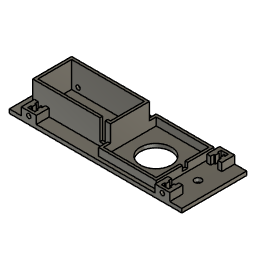
Cont Mtr Lower Case v1 (Autodesk Fusion 360 design; units mm, degrees)
Autodesk Fusion 360 part; units mm, degrees
sketch "Sketch1" plane through (0, 0, 0) normal (0, 0, 1) x (1, 0, 0)
  line L0 (0, 0) -> (60, 0)
  line L1 (60, 0) -> (60, 30)
  line L2 (60, 30) -> (0, 30)
  line L3 (0, 30) -> (0, 0)
  dimension "d1" = 60
  dimension "d2" = 30
  constraint horizontal L0
  constraint vertical L1
  constraint horizontal L2
  constraint vertical L3
  constraint coincident L0.start L3.end
  measures "d1" distance of L0.start L0.end
  measures "d2" distance of L0.start L2.end
extrude "Extrude1" add sketch "Sketch1" along normal blind 22
sketch "Sketch2" plane through (0, 0, 22) normal (0, 0, 1) x (-1, 0, 0)
  line L0 (0, -30) -> (0, 0)
  line L1 (0, 0) -> (-60, 0)
  line L2 (-60, 0) -> (-60, -30)
  line L3 (-60, -30) -> (0, -30)
  line L4 (-2, -28) -> (-58, -28)
  line L5 (-58, -28) -> (-58, -2)
  line L6 (-58, -2) -> (-2, -2)
  line L7 (-2, -2) -> (-2, -28)
  dimension "d5" = 56
  dimension "d6" = 26
  dimension "d7" = 2
  dimension "d8" = 2
  constraint horizontal L4
  constraint vertical L5
  constraint horizontal L6
  constraint vertical L7
  measures "d5" distance of L4.start L4.end
  measures "d6" distance of L4.start L6.end
  measures "d7" distance of L3 L4
  measures "d8" distance of L0 L7
extrude "Extrude2" cut sketch "Sketch2" against normal blind 20 contours L4 L5 L6 L7
sketch "Sketch3" plane through (0, 0, 0) normal (0, -1, 0) x (1, 0, 0)
  line L0 (0, 0) -> (60, 0)
  line L1 (60, 0) -> (60, 22)
  line L2 (60, 22) -> (0, 22)
  line L3 (0, 22) -> (0, 0)
  line L4 (0, 0) -> (60, 0)
  line L5 (60, 0) -> (60, 3)
  line L6 (60, 3) -> (0, 3)
  line L7 (0, 3) -> (0, 0)
  dimension "d11" = 60
  dimension "d12" = 3
  constraint horizontal L4
  constraint vertical L5
  constraint horizontal L6
  constraint vertical L7
  constraint coincident L0.start L3.end
  measures "d11" distance of L0.start L0.end
  measures "d12" distance of L0.start L6.end
extrude "Extrude3" add sketch "Sketch3" along normal blind 8 contours L0 L1 L3 L4 L5 L6 L7
sketch "Sketch4" plane through (0, 30, 0) normal (0, 1, 0) x (-1, 0, 0)
  line L0 (-60, 0) -> (0, 0)
  line L1 (0, 0) -> (0, 22)
  line L2 (0, 22) -> (-60, 22)
  line L3 (-60, 22) -> (-60, 0)
  line L4 (-60, 0) -> (0, 0)
  line L5 (0, 0) -> (0, 3)
  line L6 (0, 3) -> (-60, 3)
  line L7 (-60, 3) -> (-60, 0)
  dimension "d15" = 3
  constraint horizontal L4
  constraint vertical L5
  constraint horizontal L6
  constraint vertical L7
  constraint coincident L0.start L3.end
  measures "d15" distance of L0.start L6.end
extrude "Extrude4" add sketch "Sketch4" along normal blind 8 contours L0 L1 L3 L4 L5 L6 L7
sketch "Sketch5" plane through (60, 0, 0) normal (1, 0, 0) x (0, 1, 0)
  line L0 (-8, 0) -> (38, 0)
  line L1 (38, 0) -> (38, 3)
  line L2 (38, 3) -> (30, 3)
  line L3 (30, 3) -> (30, 22)
  line L4 (30, 22) -> (0, 22)
  line L5 (0, 22) -> (0, 3)
  line L6 (0, 3) -> (-8, 3)
  line L7 (-8, 3) -> (-8, 0)
  line L8 (-8, 3) -> (38, 3)
  line L9 (38, 3) -> (38, 0)
  line L10 (38, 0) -> (-8, 0)
  line L11 (-8, 0) -> (-8, 3)
  constraint horizontal L8
  constraint vertical L9
  constraint horizontal L10
  constraint vertical L11
  constraint coincident L0.end L1.start
  constraint coincident L6.end L7.start
extrude "Extrude5" add sketch "Sketch5" along normal blind 50 contours L0 L1 L2 L6 L7 L8 L9 L10 L11
sketch "Sketch6" plane through (0, 0, 0) normal (-1, 0, 0) x (0, -1, 0)
  line L0 (-38, 0) -> (8, 0)
  line L1 (8, 0) -> (8, 3)
  line L2 (8, 3) -> (0, 3)
  line L3 (0, 3) -> (0, 22)
  line L4 (0, 22) -> (-30, 22)
  line L5 (-30, 22) -> (-30, 3)
  line L6 (-30, 3) -> (-38, 3)
  line L7 (-38, 3) -> (-38, 0)
  line L8 (-38, 3) -> (8, 3)
  line L9 (8, 3) -> (8, 0)
  line L10 (8, 0) -> (-38, 0)
  line L11 (-38, 0) -> (-38, 3)
  constraint horizontal L8
  constraint vertical L9
  constraint horizontal L10
  constraint vertical L11
  constraint coincident L0.end L1.start
  constraint coincident L6.end L7.start
extrude "Extrude6" add sketch "Sketch6" along normal blind 8 contours L0 L1 L2 L6 L7 L8 L9 L10 L11
sketch "Sketch7" plane through (0, 0, 3) normal (0, 0, 1) x (-1, 0, 0)
  line L0 (8, 8) -> (-110, 8)
  line L1 (-110, 8) -> (-110, -38)
  line L2 (-110, -38) -> (8, -38)
  line L3 (8, -38) -> (8, 8)
  line L4 (0, 0) -> (0, -30)
  line L5 (0, -30) -> (-60, -30)
  line L6 (-60, -30) -> (-60, 0)
  line L7 (-60, 0) -> (0, 0)
  line L8 (-60.1, -35.15) -> (-100.4, -35.15) construction
  line L9 (-100.4, -35.15) -> (-100.4, 5.15) construction
  line L10 (-100.4, 5.15) -> (-60.1, 5.15) construction
  line L11 (-60.1, 5.15) -> (-60.1, -35.15) construction
  line L12 (-60, -15) -> (-127.1, -15) construction
  line L13 (-100.5, -35.25) -> (-60, -35.25)
  line L14 (-60, -35.25) -> (-60, 5.25)
  line L15 (-60, 5.25) -> (-100.5, 5.25)
  line L16 (-100.5, 5.25) -> (-100.5, -35.25)
  line L17 (-58, -37.25) -> (-58, 7.25)
  line L18 (-58, 7.25) -> (-102.5, 7.25)
  line L19 (-102.5, 7.25) -> (-102.5, -37.25)
  line L20 (-102.5, -37.25) -> (-58, -37.25)
  dimension "d22" = 40.3
  dimension "d23" = 40.3
  dimension "d24" = 20.15
  dimension "d25" = 0.1
  dimension "d31" = 40.5
  dimension "d32" = 40.5
  dimension "d33" = 68
  dimension "d34" = 20.25
  dimension "d35" = 2
  constraint horizontal L8
  constraint vertical L9
  constraint horizontal L10
  constraint vertical L11
  constraint midpoint L6 L12.start
  constraint perpendicular L1 L12
  constraint horizontal L13
  constraint vertical L14
  constraint horizontal L15
  constraint vertical L16
  measures "d22" distance of L8.start L8.end
  measures "d23" distance of L8.start L10.end
  measures "d24" distance of L8 L12
  measures "d25" distance of L6 L11
  measures "d31" distance of L13.start L13.end
  measures "d32" distance of L13.start L15.end
  measures "d33" distance of L3 L14
  measures "d34" distance of L12 L13
move_face "OffsetFaces1" offset 2 1 faces at (70.6667, 38, 2)
extrude "Extrude7" add 1 faces at (31.3333, -8, 2) along direction (0, -1, 0) blind 2
extrude "Extrude8" add 1 faces at (110, 23.3333, 1) along direction (1, 0, 0) blind 15
extrude "Extrude9" add sketch "Sketch7" along normal blind 6 contours L5 L7 L13 L14 L15 L16 L17 L18 L19 L20
sketch "Sketch9" plane through (0, 0, 3) normal (0, 0, 1) x (-1, 0, 0)
  line L0 (-60, -35.25) -> (-60, 5.25)
  line L1 (-60, 5.25) -> (-100.5, 5.25)
  line L2 (-100.5, 5.25) -> (-100.5, -35.25)
  line L3 (-100.5, -35.25) -> (-60, -35.25)
  circle A0 centre (-80, -15) radius 12
  dimension "d38" = 24
  measures "d38" diameter of A0
extrude "Extrude10" cut sketch "Sketch9" against normal blind 12 contours A0
sketch "Sketch10" plane through (0, 0, 9) normal (0, 0, 1) x (-1, 0, 0)
  line L0 (-60, 0) -> (-58, 0)
  line L1 (-58, 0) -> (-58, 7.25)
  line L2 (-58, 7.25) -> (-102.5, 7.25)
  line L3 (-102.5, 7.25) -> (-102.5, -37.25)
  line L4 (-102.5, -37.25) -> (-58, -37.25)
  line L5 (-58, -37.25) -> (-58, -30)
  line L6 (-58, -30) -> (-60, -30)
  line L7 (-60, -30) -> (-60, -35.25)
  line L8 (-60, -35.25) -> (-100.5, -35.25)
  line L9 (-100.5, -35.25) -> (-100.5, 5.25)
  line L10 (-100.5, 5.25) -> (-60, 5.25)
  line L11 (-60, 5.25) -> (-60, 0)
  line L12 (-100.5, -16.9697) -> (-102.5, -16.9697)
  line L13 (-102.5, -16.9697) -> (-102.5, -12.9697)
  line L14 (-102.5, -12.9697) -> (-100.5, -12.9697)
  line L15 (-100.5, -12.9697) -> (-100.5, -16.9697)
  line L16 (-110, -14.9697) -> (-85, -14.9697) construction
  dimension "d41" = 2
  dimension "d42" = 4
  dimension "d43" = 2
  constraint horizontal L12
  constraint vertical L13
  constraint horizontal L14
  constraint vertical L15
  constraint coincident L9 L12.start
  constraint perpendicular L9 L16
  measures "d41" distance of L12.start L12.end
  measures "d42" distance of L12.start L14.end
  measures "d43" distance of L12 L16
extrude "Extrude11" cut sketch "Sketch10" against normal blind 4 contours L3 L9 L12 L13 L14 L15
sketch "Sketch11" plane through (0, 0, 22) normal (0, 0, 1) x (-1, 0, 0)
  line L0 (-58, -28) -> (-58, -2)
  line L1 (-58, -2) -> (-2, -2)
  line L2 (-2, -2) -> (-2, -28)
  line L3 (-2, -28) -> (-58, -28)
  line L4 (0, -30) -> (0, 0)
  line L5 (0, 0) -> (-60, 0)
  line L6 (-60, 0) -> (-60, -30)
  line L7 (-60, -30) -> (0, -30)
  line L8 (-55.8802, -2) -> (-51.8802, -2)
  line L9 (-51.8802, -2) -> (-51.8802, 0)
  line L10 (-51.8802, 0) -> (-55.8802, 0)
  line L11 (-55.8802, 0) -> (-55.8802, -2)
  dimension "d46" = 4
  constraint horizontal L8
  constraint vertical L9
  constraint horizontal L10
  constraint vertical L11
  constraint coincident L1 L8.start
  measures "d46" distance of L8.start L8.end
extrude "Extrude12" cut sketch "Sketch11" against normal blind 16 contours L1 L5 L8 L9 L10 L11
sketch "Sketch12" plane through (0, 0, 3) normal (0, 0, 1) x (-1, 0, 0)
  line L0 (-58, -30) -> (-58, -37.25)
  line L1 (-58, -37.25) -> (-102.5, -37.25)
  line L2 (-102.5, -37.25) -> (-102.5, 7.25)
  line L3 (-102.5, 7.25) -> (-58, 7.25)
  line L4 (-58, 7.25) -> (-58, 0)
  line L5 (-58, 0) -> (0, 0)
  line L6 (0, 0) -> (0, -30)
  line L7 (0, -30) -> (-58, -30)
  line L8 (-125, -40) -> (8, -40)
  line L9 (8, -40) -> (8, 10)
  line L10 (8, 10) -> (-125, 10)
  line L11 (-125, 10) -> (-125, -40)
  line L12 (-7, -44) -> (-7, 24) construction
  line L13 (-110, -45) -> (-110, 22) construction
  line L14 (-1.25, -30) -> (-1.25, -40)
  line L15 (-1.25, -40) -> (-12.75, -40)
  line L16 (-12.75, -40) -> (-12.75, -30)
  line L17 (-12.75, -30) -> (-9.75, -30)
  line L18 (-9.75, -38) -> (-4.25, -38)
  line L19 (-4.25, -38) -> (-4.25, -30)
  line L20 (-1.25, -30) -> (-4.25, -30)
  line L21 (-9.75, -38) -> (-9.75, -30)
  line L22 (-28.0187, -15) -> (31, -15) construction
  line L23 (-12.75, 0) -> (-9.75, 0)
  line L24 (-12.75, 10) -> (-12.75, 0)
  line L25 (-9.75, 8) -> (-9.75, 0)
  line L26 (-9.75, 8) -> (-4.25, 8)
  line L27 (-4.25, 8) -> (-4.25, 0)
  line L28 (-1.25, 0) -> (-4.25, 0)
  line L29 (-1.25, 0) -> (-1.25, 10)
  line L30 (-1.25, 10) -> (-12.75, 10)
  line L31 (-58.5, 15) -> (-58.5, -52) construction
  line L32 (-104.25, 10) -> (-104.25, 0)
  line L33 (-115.75, 10) -> (-104.25, 10)
  line L34 (-107.25, 8) -> (-112.75, 8)
  line L35 (-107.25, 8) -> (-107.25, 0)
  line L36 (-112.75, 8) -> (-112.75, 0)
  line L37 (-115.75, 0) -> (-115.75, 10)
  line L38 (-115.75, 0) -> (-112.75, 0)
  line L39 (-104.25, 0) -> (-107.25, 0)
  line L40 (-104.25, -30) -> (-107.25, -30)
  line L41 (-107.25, -38) -> (-107.25, -30)
  line L42 (-112.75, -38) -> (-112.75, -30)
  line L43 (-115.75, -30) -> (-112.75, -30)
  line L44 (-115.75, -30) -> (-115.75, -40)
  line L45 (-107.25, -38) -> (-112.75, -38)
  line L46 (-115.75, -40) -> (-104.25, -40)
  line L47 (-104.25, -40) -> (-104.25, -30)
  dimension "d49" = 15
  dimension "d50" = 15
  dimension "d51" = 2.75
  dimension "d52" = 2.75
  dimension "d53" = 3
  dimension "d54" = 3
  dimension "d55" = 2
  dimension "d56" = 66.5
  constraint perpendicular L10 L12
  constraint perpendicular L10 L13
  constraint coincident L7 L14.start
  constraint coincident L8 L14.end
  constraint perpendicular L8 L14
  constraint coincident L8 L15.end
  constraint perpendicular L12 L15
  constraint coincident L7 L16.end
  constraint perpendicular L7 L16
  constraint coincident L7 L17.end
  constraint perpendicular L12 L18
  constraint coincident L7 L19.end
  constraint perpendicular L7 L19
  constraint perpendicular L7 L21
  constraint perpendicular L9 L22
  constraint symmetric L14.start L22 L28.start
  constraint symmetric L14.end L22 L29.end
  constraint symmetric L15.end L22 L24.start
  constraint symmetric L16.end L22 L23.start
  constraint symmetric L17.end L22 L23.end
  constraint symmetric L18.start L22 L25.start
  constraint symmetric L18.end L22 L26.end
  constraint symmetric L19.end L22 L27.end
  constraint vertical L31
  constraint symmetric L14.start L31 L43.start
  constraint symmetric L14.end L31 L44.end
  constraint symmetric L15.end L31 L46.end
  constraint symmetric L16.end L31 L40.start
  constraint symmetric L17.end L31 L40.end
  constraint symmetric L18.start L31 L41.start
  constraint symmetric L18.end L31 L42.start
  constraint symmetric L19.end L31 L42.end
  constraint symmetric L23.start L31 L32.end
  constraint symmetric L23.end L31 L35.end
  constraint symmetric L24.start L31 L32.start
  constraint symmetric L25.start L31 L34.start
  constraint symmetric L26.end L31 L34.end
  constraint symmetric L27.end L31 L36.end
  constraint symmetric L28.start L31 L37.start
  constraint symmetric L29.end L31 L33.start
  measures "d49" distance of L9 L12
  measures "d50" distance of L11 L13
  measures "d51" distance of L12 L19
  measures "d52" distance of L12 L21
  measures "d53" distance of L16 L21
  measures "d54" distance of L14 L19
  measures "d55" distance of L15 L18
  measures "d56" distance of L11 L31
extrude "Extrude13" add sketch "Sketch12" along normal blind 6 contours L7 L8 L14 L15 L16 L17 L18 L19 L20 L21 | L8 L40 L41 L42 L43 L44 L45 L46 L47 | L5 L10 L23 L24 L25 L26 L27 L28 L29 L30 | L10 L32 L33 L34 L35 L36 L37 L38 L39
sketch "Sketch13" plane through (0, -10, 0) normal (0, -1, 0) x (1, 0, 0)
  line L0 (-8, 0) -> (125, 0)
  line L1 (125, 0) -> (125, 3)
  line L2 (125, 3) -> (115.75, 3)
  line L3 (115.75, 3) -> (115.75, 9)
  line L4 (115.75, 9) -> (104.25, 9)
  line L5 (104.25, 9) -> (104.25, 3)
  line L6 (104.25, 3) -> (12.75, 3)
  line L7 (12.75, 3) -> (12.75, 9)
  line L8 (12.75, 9) -> (1.25, 9)
  line L9 (1.25, 9) -> (1.25, 3)
  line L10 (1.25, 3) -> (-8, 3)
  line L11 (-8, 3) -> (-8, 0)
  line L12 (104.25, 3) -> (115.75, 3) construction
  line L13 (103, 8.5) -> (117.6026, 8.5) construction
  line L14 (104.25, 8.5) -> (115.75, 3) construction
  line L15 (115.75, 8.5) -> (104.25, 3) construction
  line L16 (1.25, 3) -> (12.75, 3) construction
  line L17 (-3, 8.5) -> (20, 8.5) construction
  line L18 (1.25, 8.5) -> (12.75, 3) construction
  line L19 (12.75, 8.5) -> (1.25, 3) construction
  point P0 (110, 5.75)
  point P1 (7, 5.75)
  dimension "d59" = 5.5
  dimension "d60" = 5.5
  constraint coincident L5.end L6.start
  constraint coincident L2.end L3.start
  constraint perpendicular L3 L13
  constraint coincident L5 L14.start
  constraint coincident L13 L14.start
  constraint coincident L3 L15.start
  constraint coincident L13 L15.start
  constraint midpoint L15 P0
  constraint coincident L9.end L10.start
  constraint coincident L6.end L7.start
  constraint perpendicular L7 L17
  constraint coincident L9 L18.start
  constraint coincident L17 L18.start
  constraint coincident L7 L19.start
  constraint coincident L17 L19.start
  constraint midpoint L19 P1
  measures "d59" distance of L12 L13
  measures "d60" distance of L16 L17
hole "Hole1" at (7, -10, 5.75) at (110, -10, 5.75) direction (0, 1, 0) diameter 3.3 depth 100 tip angle 118
sketch "Sketch14" plane through (0, 0, 3) normal (0, 0, 1) x (-1, 0, 0)
  line L0 (-9.75, -30) -> (-9.75, -38)
  line L1 (-9.75, -38) -> (-4.25, -38)
  line L2 (-4.25, -38) -> (-4.25, -30)
  line L3 (-4.25, -30) -> (-9.75, -30)
  line L4 (-4.25, -35.5) -> (-9.75, -35.5)
  line L5 (-9.75, -35.5) -> (-9.75, -32.5)
  line L6 (-9.75, -32.5) -> (-4.25, -32.5)
  line L7 (-4.25, -32.5) -> (-4.25, -35.5)
  dimension "d64" = 3
  dimension "d65" = 2.5
  constraint horizontal L4
  constraint vertical L5
  constraint horizontal L6
  constraint vertical L7
  constraint coincident L2 L4.start
  measures "d64" distance of L4.start L6.end
  measures "d65" distance of L1 L4
extrude "Extrude14" add sketch "Sketch14" along normal blind 6 contours L0 L2 L4 L5 L6 L7
sketch "Sketch15" plane through (0, 0, 9) normal (0, 0, 1) x (-1, 0, 0)
  line L0 (-4.25, -35.5) -> (-4.25, -38)
  line L1 (-4.25, -38) -> (-9.75, -38)
  line L2 (-9.75, -38) -> (-9.75, -35.5)
  line L3 (-9.75, -35.5) -> (-4.25, -35.5)
  line L4 (-4.25, -32.5) -> (-9.75, -32.5)
  line L5 (-9.75, -32.5) -> (-9.75, -30)
  line L6 (-9.75, -30) -> (-12.75, -30)
  line L7 (-12.75, -30) -> (-12.75, -40)
  line L8 (-12.75, -40) -> (-1.25, -40)
  line L9 (-1.25, -40) -> (-1.25, -30)
  line L10 (-1.25, -30) -> (-4.25, -30)
  line L11 (-4.25, -30) -> (-4.25, -32.5)
  line L12 (-7, -25.2955) -> (-7, -46) construction
  line L13 (-5.3, -35.5) -> (-8.7, -35.5)
  line L14 (-8.7, -35.5) -> (-8.7, -32.5)
  line L15 (-8.7, -32.5) -> (-5.3, -32.5)
  line L16 (-5.3, -32.5) -> (-5.3, -35.5)
  dimension "d68" = 3.4
  dimension "d69" = 1.7
  dimension "d70" = 5.75
  constraint perpendicular L8 L12
  constraint horizontal L13
  constraint vertical L14
  constraint horizontal L15
  constraint vertical L16
  constraint coincident L3 L13.start
  measures "d68" distance of L13.start L13.end
  measures "d69" distance of L12 L14
  measures "d70" distance of L9 L12
extrude "Extrude15" cut sketch "Sketch15" against normal blind 6 contours L3 L4 L13 L14 L15 L16
sketch "Sketch16" plane through (0, 0, 3) normal (0, 0, 1) x (-1, 0, 0)
  line L0 (-9.75, 8) -> (-9.75, 0)
  line L1 (-9.75, 0) -> (-4.25, 0)
  line L2 (-4.25, 0) -> (-4.25, 8)
  line L3 (-4.25, 8) -> (-9.75, 8)
  line L4 (-7, 2) -> (-7, 16) construction
  line L5 (-1.25, 0) -> (-1.25, 10) construction
  line L6 (-4.25, 2.5) -> (-9.75, 2.5)
  line L7 (-9.75, 2.5) -> (-9.75, 5.5)
  line L8 (-9.75, 5.5) -> (-4.25, 5.5)
  line L9 (-4.25, 5.5) -> (-4.25, 2.5)
  dimension "d73" = 5.75
  dimension "d74" = 3
  dimension "d75" = 2.5
  constraint perpendicular L3 L4
  constraint horizontal L6
  constraint vertical L7
  constraint horizontal L8
  constraint vertical L9
  constraint coincident L2 L6.start
  measures "d73" distance of L4 L5
  measures "d74" distance of L6.start L8.end
  measures "d75" distance of L3 L8
extrude "Extrude16" add sketch "Sketch16" along normal blind 6 contours L0 L2 L6 L7 L8 L9
sketch "Sketch17" plane through (0, 0, 9) normal (0, 0, 1) x (-1, 0, 0)
  line L0 (-4.25, 2.5) -> (-4.25, 0)
  line L1 (-4.25, 0) -> (-1.25, 0)
  line L2 (-1.25, 0) -> (-1.25, 10)
  line L3 (-1.25, 10) -> (-12.75, 10)
  line L4 (-12.75, 10) -> (-12.75, 0)
  line L5 (-12.75, 0) -> (-9.75, 0)
  line L6 (-9.75, 0) -> (-9.75, 2.5)
  line L7 (-9.75, 2.5) -> (-4.25, 2.5)
  line L8 (-4.25, 5.5) -> (-9.75, 5.5)
  line L9 (-9.75, 5.5) -> (-9.75, 8)
  line L10 (-9.75, 8) -> (-4.25, 8)
  line L11 (-4.25, 8) -> (-4.25, 5.5)
  line L12 (-7, 1) -> (-7, 15) construction
  line L13 (-5.3, 2.5) -> (-8.7, 2.5)
  line L14 (-8.7, 2.5) -> (-8.7, 5.5)
  line L15 (-8.7, 5.5) -> (-5.3, 5.5)
  line L16 (-5.3, 5.5) -> (-5.3, 2.5)
  dimension "d78" = 5.75
  dimension "d79" = 3.4
  dimension "d80" = 1.7
  constraint perpendicular L7 L12
  constraint horizontal L13
  constraint vertical L14
  constraint horizontal L15
  constraint vertical L16
  constraint coincident L7 L13.start
  measures "d78" distance of L2 L12
  measures "d79" distance of L13.start L13.end
  measures "d80" distance of L12 L14
extrude "Extrude17" cut sketch "Sketch17" against normal blind 6 contours L7 L8 L13 L14 L15 L16
sketch "Sketch18" plane through (0, 0, 3) normal (0, 0, 1) x (-1, 0, 0)
  line L0 (-12.75, -40) -> (-12.75, -30)
  line L1 (-12.75, -30) -> (-58, -30)
  line L2 (-58, -30) -> (-58, -37.25)
  line L3 (-58, -37.25) -> (-102.5, -37.25)
  line L4 (-102.5, -37.25) -> (-102.5, 7.25)
  line L5 (-102.5, 7.25) -> (-58, 7.25)
  line L6 (-58, 7.25) -> (-58, 0)
  line L7 (-58, 0) -> (-12.75, 0)
  line L8 (-12.75, 0) -> (-12.75, 10)
  line L9 (-12.75, 10) -> (-104.25, 10)
  line L10 (-104.25, 10) -> (-104.25, 0)
  line L11 (-104.25, 0) -> (-107.25, 0)
  line L12 (-107.25, 0) -> (-107.25, 8)
  line L13 (-107.25, 8) -> (-112.75, 8)
  line L14 (-112.75, 8) -> (-112.75, 0)
  line L15 (-112.75, 0) -> (-115.75, 0)
  line L16 (-115.75, 0) -> (-115.75, 10)
  line L17 (-115.75, 10) -> (-125, 10)
  line L18 (-125, 10) -> (-125, -40)
  line L19 (-125, -40) -> (-115.75, -40)
  line L20 (-115.75, -40) -> (-115.75, -30)
  line L21 (-115.75, -30) -> (-112.75, -30)
  line L22 (-112.75, -30) -> (-112.75, -38)
  line L23 (-112.75, -38) -> (-107.25, -38)
  line L24 (-107.25, -38) -> (-107.25, -30)
  line L25 (-107.25, -30) -> (-104.25, -30)
  line L26 (-104.25, -30) -> (-104.25, -40)
  line L27 (-104.25, -40) -> (-12.75, -40)
  line L28 (-107.25, -35.5) -> (-112.75, -35.5)
  line L29 (-112.75, -35.5) -> (-112.75, -32.5)
  line L30 (-112.75, -32.5) -> (-107.25, -32.5)
  line L31 (-107.25, -32.5) -> (-107.25, -35.5)
  line L32 (-107.25, 2.5) -> (-112.75, 2.5)
  line L33 (-112.75, 2.5) -> (-112.75, 5.5)
  line L34 (-112.75, 5.5) -> (-107.25, 5.5)
  line L35 (-107.25, 5.5) -> (-107.25, 2.5)
  dimension "d83" = 3
  dimension "d84" = 3
  dimension "d85" = 2.5
  dimension "d86" = 2.5
  constraint horizontal L28
  constraint vertical L29
  constraint horizontal L30
  constraint vertical L31
  constraint coincident L24 L28.start
  constraint horizontal L32
  constraint vertical L33
  constraint horizontal L34
  constraint vertical L35
  constraint coincident L12 L32.start
  measures "d83" distance of L28.start L30.end
  measures "d84" distance of L32.start L34.end
  measures "d85" distance of L23 L28
  measures "d86" distance of L13 L34
extrude "Extrude18" add sketch "Sketch18" along normal blind 6 contours L22 L24 L28 L29 L30 L31 | L12 L14 L32 L33 L34 L35
sketch "Sketch19" plane through (0, 0, 9) normal (0, 0, 1) x (-1, 0, 0)
  line L0 (-112.75, -32.5) -> (-112.75, -30)
  line L1 (-112.75, -30) -> (-115.75, -30)
  line L2 (-115.75, -30) -> (-115.75, -40)
  line L3 (-115.75, -40) -> (-104.25, -40)
  line L4 (-104.25, -40) -> (-104.25, -30)
  line L5 (-104.25, -30) -> (-107.25, -30)
  line L6 (-107.25, -30) -> (-107.25, -32.5)
  line L7 (-107.25, -32.5) -> (-112.75, -32.5)
  line L8 (-112.75, -35.5) -> (-107.25, -35.5)
  line L9 (-107.25, -35.5) -> (-107.25, -38)
  line L10 (-107.25, -38) -> (-112.75, -38)
  line L11 (-112.75, -38) -> (-112.75, -35.5)
  line L12 (-108.3, -35.5) -> (-111.7, -35.5)
  line L13 (-111.7, -35.5) -> (-111.7, -32.5)
  line L14 (-111.7, -32.5) -> (-108.3, -32.5)
  line L15 (-108.3, -32.5) -> (-108.3, -35.5)
  line L16 (-110, -40.7377) -> (-110, -29.5) construction
  dimension "d89" = 3.4
  dimension "d90" = 5.75
  dimension "d91" = 1.7
  constraint horizontal L12
  constraint vertical L13
  constraint horizontal L14
  constraint vertical L15
  constraint coincident L8 L12.start
  constraint perpendicular L7 L16
  measures "d89" distance of L12.start L12.end
  measures "d90" distance of L2 L16
  measures "d91" distance of L13 L16
extrude "Extrude19" cut sketch "Sketch19" against normal blind 6 contours L7 L8 L12 L13 L14 L15
sketch "Sketch20" plane through (0, 0, 9) normal (0, 0, 1) x (-1, 0, 0)
  line L0 (-112.75, 5.5) -> (-112.75, 8)
  line L1 (-112.75, 8) -> (-107.25, 8)
  line L2 (-107.25, 8) -> (-107.25, 5.5)
  line L3 (-107.25, 5.5) -> (-112.75, 5.5)
  line L4 (-112.75, 2.5) -> (-107.25, 2.5)
  line L5 (-107.25, 2.5) -> (-107.25, 0)
  line L6 (-107.25, 0) -> (-104.25, 0)
  line L7 (-104.25, 0) -> (-104.25, 10)
  line L8 (-104.25, 10) -> (-115.75, 10)
  line L9 (-115.75, 10) -> (-115.75, 0)
  line L10 (-115.75, 0) -> (-112.75, 0)
  line L11 (-112.75, 0) -> (-112.75, 2.5)
  line L12 (-108.2353, 2.5) -> (-111.6353, 2.5)
  line L13 (-111.6353, 2.5) -> (-111.6353, 5.5)
  line L14 (-111.6353, 5.5) -> (-108.2353, 5.5)
  line L15 (-108.2353, 5.5) -> (-108.2353, 2.5)
  line L16 (-109.9353, -2) -> (-109.9353, 11) construction
  dimension "d94" = 3.4
  dimension "d95" = 1.7
  constraint horizontal L12
  constraint vertical L13
  constraint horizontal L14
  constraint vertical L15
  constraint coincident L4 L12.start
  constraint perpendicular L8 L16
  measures "d94" distance of L12.start L12.end
  measures "d95" distance of L13 L16
extrude "Extrude20" cut sketch "Sketch20" against normal blind 6 contours L3 L4 L12 L13 L14 L15
sketch "Sketch21" plane through (0, 0, 3) normal (0, 0, 1) x (-1, 0, 0)
  line L0 (-107.25, -35.5) -> (-108.3, -35.5)
  line L1 (-108.3, -35.5) -> (-108.3, -32.5)
  line L2 (-108.3, -32.5) -> (-107.25, -32.5)
  line L3 (-107.25, -32.5) -> (-107.25, -30)
  line L4 (-107.25, -30) -> (-104.25, -30)
  line L5 (-104.25, -30) -> (-104.25, -40)
  line L6 (-104.25, -40) -> (-12.75, -40)
  line L7 (-12.75, -40) -> (-12.75, -30)
  line L8 (-12.75, -30) -> (-58, -30)
  line L9 (-58, -30) -> (-58, -37.25)
  line L10 (-58, -37.25) -> (-102.5, -37.25)
  line L11 (-102.5, -37.25) -> (-102.5, 7.25)
  line L12 (-102.5, 7.25) -> (-58, 7.25)
  line L13 (-58, 7.25) -> (-58, 0)
  line L14 (-58, 0) -> (-12.75, 0)
  line L15 (-12.75, 0) -> (-12.75, 10)
  line L16 (-12.75, 10) -> (-104.25, 10)
  line L17 (-104.25, 10) -> (-104.25, 0)
  line L18 (-104.25, 0) -> (-107.25, 0)
  line L19 (-107.25, 0) -> (-107.25, 2.5)
  line L20 (-107.25, 2.5) -> (-108.2353, 2.5)
  line L21 (-108.2353, 2.5) -> (-108.2353, 5.5)
  line L22 (-108.2353, 5.5) -> (-107.25, 5.5)
  line L23 (-107.25, 5.5) -> (-107.25, 8)
  line L24 (-107.25, 8) -> (-112.75, 8)
  line L25 (-112.75, 8) -> (-112.75, 5.5)
  line L26 (-112.75, 5.5) -> (-111.6353, 5.5)
  line L27 (-111.6353, 5.5) -> (-111.6353, 2.5)
  line L28 (-111.6353, 2.5) -> (-112.75, 2.5)
  line L29 (-112.75, 2.5) -> (-112.75, 0)
  line L30 (-112.75, 0) -> (-115.75, 0)
  line L31 (-115.75, 0) -> (-115.75, 10)
  line L32 (-115.75, 10) -> (-125, 10)
  line L33 (-125, 10) -> (-125, -40)
  line L34 (-125, -40) -> (-115.75, -40)
  line L35 (-115.75, -40) -> (-115.75, -30)
  line L36 (-115.75, -30) -> (-112.75, -30)
  line L37 (-112.75, -30) -> (-112.75, -32.5)
  line L38 (-112.75, -32.5) -> (-111.7, -32.5)
  line L39 (-111.7, -32.5) -> (-111.7, -35.5)
  line L40 (-111.7, -35.5) -> (-112.75, -35.5)
  line L41 (-112.75, -35.5) -> (-112.75, -38)
  line L42 (-112.75, -38) -> (-107.25, -38)
  line L43 (-107.25, -38) -> (-107.25, -35.5)
  line L44 (-102.5, -15) -> (-131, -15) construction
  point P0 (-112.5, -15)
  dimension "d98" = 10
  constraint midpoint L11 L44.start
  constraint perpendicular L33 L44
  constraint coincident L44 P0
  measures "d98" distance of L11 P0
hole "Hole2" at (112.5, 15, 3) direction (0, 0, -1) diameter 5.3 depth 100 tip angle 118
